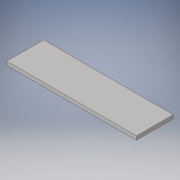
# Autodesk Inventor part: aLMOST uSELESS pART!!
Saved by Autodesk Inventor 2016 (Build 200138000, 138)
## iProperties
Created: 2017-01-31
Part Number: aLMOST uSELESS pART!!
Material: Generic
Document SubType Name: Modeling
Designer: student1
Density: 1 g/cm^3
Appearance: Default
Mass: 5.76169 g
Surface Area: 51.1947 cm^2
Volume: 5.76169 cm^3
Author: student1
Autodesk Inventor part; units mm, degrees
ref_plane "YZ Plane" through (0, 0, 0) normal (1, 0, 0) x (0, 1, 0)
ref_plane "XZ Plane" through (0, 0, 0) normal (0, 1, 0) x (-1, 0, 0)
ref_plane "XY Plane" through (0, 0, 0) normal (0, 0, 1) x (1, 0, 0)
sketch "Sketch1" plane through (0, 0, 0) normal (0, 1, 0) x (-1, 0, 0)
  line L0 (53.5517, 20.7433) -> (-35.7547, 20.7433)
  line L1 (-35.7547, 20.7433) -> (-35.7547, -4.6567)
  line L2 (-35.7547, -4.6567) -> (53.5517, -4.6567)
  line L3 (53.5517, -4.6567) -> (53.5517, 20.7433)
  point P0 (0, 0)
  dimension "d0" = 25.4
  dimension "d1" = 89.3064
  constraints: 8 end point, 2 parallel, 1 horizontal, 1 perpendicular
  measures "d0" distance of L2.end L0.start
  measures "d1" distance of L1.end L2.end
extrude "Extrusion1" add sketch "Sketch1" along normal blind 2.54
body "Solid1"
